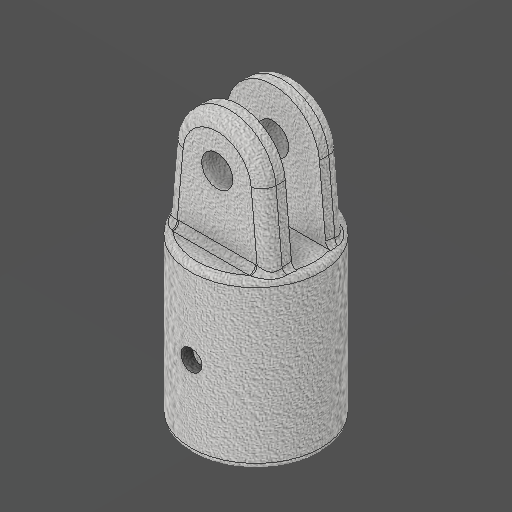
# Autodesk Inventor part: LF50-6
Saved by Autodesk Inventor 2021 (Build 250183000, 183)
## iProperties
Created: 2020-04-23
Part Number: LF50-6
Material: Aluminium Cast
Document SubType Name: Modeling
Designer: Hannah
Density: 4.2402 g/cm^3
Appearance: Aluminum Cast
Mass: 170 g
Surface Area: 196.194 cm^2
Volume: 40.0924 cm^3
Vendor: Kee Systems
Description: female swivel socket
Catalog Web Link: https://keesystems.com/store/fittings/kee-lite/lf50-female-single-swivel-socket-member.html
Size: 6
Author: Hannah
Revision Number: -
Autodesk Inventor part; units mm, degrees
ref_plane "YZ Plane" through (0, 0, 0) normal (1, 0, 0) x (0, 1, 0)
ref_plane "XZ Plane" through (0, 0, 0) normal (0, 1, 0) x (-1, 0, 0)
ref_plane "XY Plane" through (0, 0, 0) normal (0, 0, 1) x (1, 0, 0)
sketch "Sketch2" plane through (0, 0, 0) normal (0, 1, 0) x (-1, 0, 0)
  circle A0 centre (0, 0) radius 17.5
  circle A1 centre (0, 0) radius 21
  dimension "d5" = 35
  dimension "d6" = 42
  constraints: 2 centre point, 2 coincident
  measures "d5" diameter of A0
  measures "d6" diameter of A1
extrude "Extrusion2" add sketch "Sketch2" along normal mid plane 53 contours A0 | A1
extrude "Extrusion3" cut sketch "Sketch2" along normal blind 21.5 and the other way blind 26.5 contours A0
hole "Hole1" at (0, 0, 0) direction (0, 0, 1) diameter 6.647 end through all thread size "M8x1.25" class "6H" standard "ISO Metric profile"
sketch "Sketch3" plane through (0, 0, 0) normal (0, 0, 1) x (1, 0, 0)
  circle A0 centre (0, 48.5) radius 5
  arc A1 (14.9392, 49.8495) -> (-14.9392, 49.8495) centre (0, 48.5) ccw
  line L0 (-17.0483, 26.5) -> (-14.9392, 49.8495)
  line L1 (14.9392, 49.8495) -> (17.0483, 26.5)
  line L2 (17.5, 21.5) -> (-17.5, 21.5) projected
  line L3 (-21, -26.5) -> (21, -26.5) projected
  line L4 (21, 26.5) -> (-21, 26.5) projected
  line L5 (-17.0483, 26.5) -> (17.0483, 26.5)
  point P0 (0, 0)
  dimension "d36" = 10
  dimension "d37" = 15
  dimension "d50" = 75
  constraints: 6 end point, 4 point on line, 2 centre point, 2 point on circle, 2 tangent, 1 coincident, 1 equal length
  measures "d36" diameter of A0
  measures "d37" radius of A1
  measures "d50" distance from line of L3 A0.centre
extrude "Extrusion5" add sketch "Sketch3" along normal mid plane 25
extrude "Extrusion6" cut sketch "Sketch3" along normal mid plane 11
fillet "Fillet2" radius 4 6 edges at (0, 63.5, 12.5) (15.9938, 38.1747, 12.5) (-15.9938, 38.1747, 12.5) (0, 63.5, -12.5) (15.9938, 38.1747, -12.5) (-15.9938, 38.1747, -12.5)
fillet "Fillet2" radius 2 10 edges at (0, 26.5, 21) (-16.9619, 26.5, 12.3812) (16.9619, 26.5, 12.3812) (21, 26.5, 0) (-16.9619, 26.5, -12.3812) (16.9619, 26.5, -12.3812) (0, 26.5, -21) (-19.9877, 26.5, -6.4415) (-19.9877, 26.5, 6.4415) (21, -26.5, 0)
fillet "Fillet3" radius 2 7 edges at (-13.816, 26.5, 12.4231) (14.5697, 26.5, 12.1952) (13.816, 26.5, 12.4231) (0, 26.5, 12.5) (13.8156, 26.5, -12.4231) (0, 26.5, -12.5) (-13.816, 26.5, -12.4231)
equation "\"d46\" = 0.5 * d7"
equation "\"d7\" = 53"
body "Solid1"
